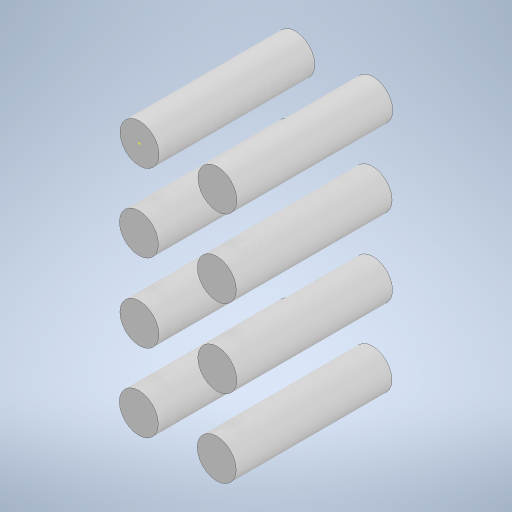
# Autodesk Inventor part: WRO Modell_RC_Auto_4
Saved by Autodesk Inventor 2024 (Build 280153000, 153)
## iProperties
Created: 2025-03-13
Part Number: WRO Modell_RC_Auto_4
Material: Generisch
Document SubType Name: Modeling
Designer: SFZ7-PC
Density: 1 g/cm^3
Appearance: Vorgabe
Author: SFZ7-PC
Autodesk Inventor part; units mm, degrees
ref_plane "YZ Plane" through (0, 0, 0) normal (1, 0, 0) x (0, 1, 0)
ref_plane "XZ Plane" through (0, 0, 0) normal (0, 1, 0) x (-1, 0, 0)
ref_plane "XY Plane" through (0, 0, 0) normal (0, 0, 1) x (1, 0, 0)
sketch "Skizze1" plane through (0, 0, 0) normal (0, 1, 0) x (-1, 0, 0)
  point P0 (0, 0)
sketch "Skizze31" plane through (0, 0, 0) normal (0, 1, 0) x (-1, 0, 0)
  circle A0 centre (0, 0) radius 2.5
  circle A1 centre (-10, -0.072) radius 2.5
  circle A2 centre (0.0751, -10) radius 2.5
  circle A3 centre (-9.9249, -10.072) radius 2.5
  circle A4 centre (0.0145, -20) radius 2.5
  circle A5 centre (-9.9855, -20.072) radius 2.5
  circle A6 centre (0.0896, -30) radius 2.5
  circle A7 centre (-9.9104, -30.072) radius 2.5
  dimension "d186" = 5
  dimension "d187" = 5
  dimension "d188" = 10
  dimension "d189" = 5
  dimension "d190" = 5
  dimension "d191" = 10
  dimension "d192" = 10
  dimension "d193" = 5
  dimension "d194" = 5
  dimension "d195" = 10
  dimension "d196" = 5
  dimension "d197" = 5
  dimension "d198" = 10
  dimension "d199" = 10
  dimension "d200" = 10
  constraints: 8 centre point, 8 coincident
  measures "d186" diameter of A0
  measures "d187" diameter of A1
  measures "d188" horizontal distance of point (-10, -0.072) point (0, 0)
  measures "d189" diameter of A2
  measures "d190" diameter of A3
  measures "d191" horizontal distance of point (-9.925, -10.072) point (0.075, -10)
  measures "d192" vertical distance of point (0.075, -10) point (0, 0)
  measures "d193" diameter of A4
  measures "d194" diameter of A5
  measures "d195" horizontal distance of point (-9.986, -20.072) point (0.014, -20)
  measures "d196" diameter of A6
  measures "d197" diameter of A7
  measures "d198" horizontal distance of point (-9.91, -30.072) point (0.09, -30)
  measures "d199" vertical distance of point (0.09, -30) point (0.014, -20)
  measures "d200" vertical distance of point (0.014, -20) A2.centre
extrude "Extrusion21" add sketch "Skizze31" along normal blind 20
